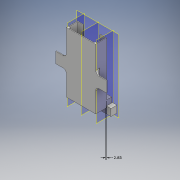
# Autodesk Inventor part: battery_case_1
Saved by Autodesk Inventor 2018 (Build 220112000, 112)
## iProperties
Created: 2019-07-20
Part Number: battery_case_1
Material: 一般
Document SubType Name: Modeling
Designer: guest1
Density: 1 g/cm^3
Appearance: 既定
Author: guest1
Autodesk Inventor part; units mm, degrees
ref_plane "YZ Plane" through (0, 0, 0) normal (1, 0, 0) x (0, 1, 0)
sketch "スケッチ1" plane through (0, 0, 0) normal (0, 0, 1) x (1, 0, 0)
  line L0 (-42.125, -17.075) -> (42.125, -17.075)
  line L1 (42.125, -17.075) -> (42.125, 15.125)
  line L2 (42.125, 15.125) -> (-42.125, 15.125)
  line L3 (-42.125, 15.125) -> (-42.125, -17.075)
  point P0 (0, 0)
  dimension "d0" = 84.25
  dimension "d1" = 32.2
  dimension "d140" = 15.125
  constraints: 8 end point, 2 parallel, 1 horizontal, 1 perpendicular
  measures "d0" distance of L1.end L2.end
  measures "d1" distance of L2.end L0.start
  measures "d140" distance from line of point (0, 0) L2
extrude "本体＿側" add sketch "スケッチ1" against normal blind 174
sketch "スケッチ3" plane through (0, 0, 0) normal (0, 0, 1) x (1, 0, 0)
  line L0 (-40.125, -12.075) -> (40.125, -12.075)
  line L1 (40.125, -12.075) -> (40.125, 13.125)
  line L2 (40.125, 13.125) -> (-40.125, 13.125)
  line L3 (-40.125, 13.125) -> (-40.125, -12.075)
  line L4 (42.125, 15.125) -> (-42.125, 15.125) projected
  line L5 (-42.125, -17.075) -> (42.125, -17.075) projected
  line L6 (-42.125, 15.125) -> (-42.125, -17.075) projected
  dimension "d4" = 80.25
  dimension "d125" = 2
  dimension "d138" = 2
  dimension "d139" = 25.2
  constraints: 8 end point, 2 parallel, 1 horizontal, 1 perpendicular
  measures "d4" distance of L1.end L2.end
  measures "d125" distance from line of L4 L2.end
  measures "d138" distance between parallel lines of L6 L3
  measures "d139" distance of L2.end L0.start
extrude "本体" cut sketch "スケッチ3" against normal blind 170
sketch "スケッチ6" plane through (0, 0, -174) normal (0, 0, -1) x (-1, 0, 0)
  line L0 (55, 48.1251) -> (-55, 48.1251)
  line L1 (-55, 48.1251) -> (-55, 14.1251)
  line L2 (-55, 14.1251) -> (55, 14.1251)
  line L3 (55, 14.1251) -> (55, 48.1251)
  line L4 (55, 48.1251) -> (-55, 14.1251) construction
  line L5 (-55, 48.1251) -> (55, 14.1251) construction
  line L6 (0, 0) -> (0, 97.4837)
  point P0 (0, 31.1251)
  point P1 (0, 31.1251)
  dimension "d8" = 110
  dimension "d9" = 34
  constraints: 14 end point, 3 midpoint, 3 parallel, 1 horizontal, 1 perpendicular, 1 point on line
  measures "d8" distance of L0.start L0.end
  measures "d9" distance of L0.end L1.end
extrude "カメラ" add sketch "スケッチ6" along normal blind 15.5 and the other way blind 4.5
sketch "スケッチ7" plane through (0, 0, -189.5) normal (0, 0, -1) x (-1, 0, 0)
  line L0 (-55, 48.1251) -> (-55, 14.1251) projected
  line L1 (-53, 16.1124) -> (53, 16.1124)
  line L2 (53, 16.1124) -> (53, 46.2624)
  line L3 (53, 46.2624) -> (-53, 46.2624)
  line L4 (-53, 46.2624) -> (-53, 16.1124)
  line L5 (-53, 16.1124) -> (53, 46.2624) construction
  line L6 (53, 16.1124) -> (-53, 46.2624) construction
  point P0 (0, 0)
  point P1 (-55, 31.1251)
  point P2 (-55, 31.1251)
  point P3 (0, 31.1874)
  point P4 (0, 31.1874)
  dimension "d14" = 30.15
  dimension "d15" = 106
  constraints: 12 end point, 4 midpoint, 2 parallel, 1 coincident, 1 horizontal, 1 perpendicular, 1 other
  measures "d14" distance of L1.end L2.end
  measures "d15" distance of L2.end L3.end
extrude "カメラ＿本体" cut sketch "スケッチ7" against normal blind 18
ref_plane "作業平面1" through (-55, 31.1251, -189.5) normal (0, 1, 0) x (1, 0, 0)
ref_plane "作業平面2" through (0, 14.1251, -189.5) normal (-1, 0, 0) x (0, 0, 1)
sketch "スケッチ10" plane through (-53, 16.1124, -189.5) normal (0, 1, 0) x (1, 0, 0)
  line L0 (59.8, -12.45) -> (46.2, -12.45)
  line L1 (46.2, -12.45) -> (46.2, 0)
  line L2 (46.2, 0) -> (59.8, 0)
  line L3 (59.8, 0) -> (59.8, -12.45)
  line L4 (59.8, -12.45) -> (46.2, 0) construction
  line L5 (46.2, -12.45) -> (59.8, 0) construction
  line L6 (108, -20) -> (-2, -20)
  line L7 (53, -20) -> (53, -4.9349)
  line L8 (53, -227.4) -> (53, 37.9)
  line L9 (0, 0) -> (106, 0)
  line L10 (0, 0) -> (106, 0)
  line L11 (0, 0) -> (0, -18)
  line L12 (0, -18) -> (106, -18)
  line L13 (106, 0) -> (106, -18)
  point P0 (53, -189.5)
  point P1 (53, -6.225)
  point P2 (53, 0)
  dimension "d22" = 12.45
  dimension "d23" = 13.6
  constraints: 28 end point, 4 midpoint, 1 point on line
  measures "d22" distance of L0.end L1.end
  measures "d23" distance of L0.start L0.end
sketch "スケッチ11" plane through (0, 0, -169.5) normal (0, 0, 1) x (1, 0, 0)
  line L0 (-15, 22.8501) -> (15, 22.8501)
  line L1 (15, 22.8501) -> (15, 39.4001)
  line L2 (15, 39.4001) -> (-15, 39.4001)
  line L3 (-15, 39.4001) -> (-15, 22.8501)
  line L4 (-53, 31.1251) -> (53, 31.1251)
  line L5 (-15, 22.8501) -> (15, 39.4001) construction
  line L6 (15, 22.8501) -> (-15, 39.4001) construction
  line L7 (0, -24.4525) -> (0, 47.8399)
  point P0 (0, 0)
  point P1 (0, 31.1251)
  point P2 (0, 31.1251)
  dimension "d26" = 30
  dimension "d27" = 16.55
  constraints: 16 end point, 4 midpoint, 1 point on line
  measures "d26" distance of L1.end L2.end
  measures "d27" distance of L2.end L0.start
extrude "突起" cut sketch "スケッチ10" against normal blind 2 contours L0 L7 L8 L2 L3 | L0 L1 L2 L8 L7
extrude "コード" cut sketch "スケッチ11" against normal blind 2
ref_plane "作業平面6" through (53, 16.1124, -189.5) normal (0, 0, 1) x (1, 0, 0)
sketch "スケッチ18" plane through (53, 16.1124, -189.5) normal (0, 0, 1) x (1, 0, 0)
  line L0 (0, 0) -> (0, 30.15) projected
  ellipse E0 centre (0, 15.0748) end of major axis (0, 0) minor radius 3.8117 (0, 30.1495) -> (0, 0) ccw
  line L1 (0, 30.15) -> (-106, 30.15) projected
  line L2 (-106, 0) -> (0, 0) projected
  line L3 (0, 30.15) -> (0, 0)
  point P0 (-53, -16.1124)
  constraints: 3 end point, 2 point on line, 2 vertical, 4 other
extrude "半円１" add sketch "スケッチ18" along normal blind 2
sketch "スケッチ19" plane through (53, 16.1124, -189.5) normal (0, 0, 1) x (1, 0, 0)
  line L0 (-106, 30.15) -> (-106, 0) projected
  ellipse E0 centre (-106.01, 15.0751) end of major axis (-106.0154, 30.1501) minor radius 3.8117 (-106.01, 0) -> (-106.01, 30.1501) ccw
  line L1 (-38, 6.7377) -> (-38, 23.2877) projected
  line L2 (-38, 23.2877) -> (-68, 23.2877) projected
  line L3 (-68, 23.2877) -> (-68, 6.7377) projected
  line L4 (-68, 6.7377) -> (-38, 6.7377) projected
  line L5 (-106, 0) -> (0, 0) projected
  line L6 (-106, 30.15) -> (-106, 0) projected
  line L7 (0, 30.15) -> (-106, 30.15) projected
  line L8 (0, 0) -> (0, 30.15) projected
  line L9 (-106, 0) -> (0, 0) projected
  line L10 (0, 30.15) -> (-106, 30.15) projected
  line L11 (-106, 0) -> (-106, 30.15)
  point P0 (-53, -16.1124)
  constraints: 2 end point, 1 perpendicular, 6 other
extrude "半円2" add sketch "スケッチ19" along normal blind 2 contours E0 L0
sketch "スケッチ16" plane through (-55, 31.1251, -189.5) normal (0, 1, 0) x (1, 0, 0)
  line L0 (110, -20) -> (110, 0) projected
  line L1 (0, -20) -> (0, 0) projected
  line L2 (110, 0) -> (0, 0)
  line L3 (0, 0) -> (0, -20)
  line L4 (0, -20) -> (110, -20)
  line L5 (110, -20) -> (110, 0)
  point P0 (55, -189.5)
  constraints: 8 end point, 2 parallel, 1 horizontal, 1 perpendicular
extrude "上半分消去" cut sketch "スケッチ16" along normal blind 17
sketch "スケッチ20" plane through (-42.125, 15.125, 0) normal (0, 1, 0) x (1, 0, 0)
  line L0 (18, 0) -> (66.25, 0)
  line L1 (66.25, 0) -> (66.25, 170)
  line L2 (66.25, 170) -> (18, 170)
  line L3 (18, 170) -> (18, 0)
  line L4 (18, 0) -> (66.25, 170) construction
  line L5 (66.25, 0) -> (18, 170) construction
  line L6 (84.25, 0) -> (0, 0) projected
  line L7 (42.125, -37.9) -> (42.125, 227.4) projected
  point P0 (42.125, 85)
  point P1 (42.125, 0)
  point P2 (42.125, 85)
  dimension "d47" = 170
  dimension "d91" = 18
  constraints: 12 end point, 5 midpoint, 3 coincident, 2 parallel, 1 horizontal, 1 perpendicular, 1 point on line
  measures "d47" distance of L2.end L0.start
  measures "d91" distance of L6.start L0.end
extrude "ボタン部" cut sketch "スケッチ20" against normal blind 2
ref_plane "作業平面7" through (-42.125, 15.125, 0) normal (-1, 0, 0) x (0, 0, -1)
sketch "スケッチ22" plane through (-42.125, 15.125, 0) normal (-1, 0, 0) x (0, 0, -1)
  line L0 (0, 0) -> (174, 0) projected
  line L1 (169.5, 0) -> (154.5, 0)
  line L2 (154.5, 0) -> (154.5, -14)
  line L3 (154.5, -14) -> (169.5, -14)
  line L4 (169.5, -14) -> (169.5, 0)
  point P0 (0, 15.125)
  point P1 (169.5, 0.9999)
  dimension "d51" = 15
  dimension "d52" = 14
  constraints: 8 end point, 2 parallel, 2 point on line, 1 horizontal, 1 perpendicular
  measures "d51" distance of L2.end L3.end
  measures "d52" distance of L1.end L2.end
extrude "支え１" add sketch "スケッチ22" against normal blind 15
ref_plane "作業平面8" through (42.125, 15.125, 0) normal (-1, 0, 0) x (0, 0, -1)
sketch "スケッチ23" plane through (42.125, 15.125, 0) normal (-1, 0, 0) x (0, 0, -1)
  line L0 (0, 0) -> (174, 0) projected
  line L1 (154.5, -14) -> (154.5, 0) projected
  line L2 (169.5, 0) -> (154.5, 0)
  line L3 (154.5, 0) -> (154.5, -14)
  line L4 (154.5, -14) -> (169.5, -14)
  line L5 (169.5, -14) -> (169.5, 0)
  point P0 (0, 15.125)
  dimension "d55" = 15
  dimension "d56" = 14
  constraints: 8 end point, 2 parallel, 1 horizontal, 1 perpendicular, 1 point on line
  measures "d55" distance of L1.start L4.end
  measures "d56" distance of L1.start L1.end
extrude "支え２" add sketch "スケッチ23" along normal blind 15
ref_plane "作業平面9" through (42.125, -17.075, 0) normal (0, 0, 1) x (0, 1, 0)
sketch "スケッチ24" plane through (42.125, -17.075, 0) normal (0, 0, 1) x (0, 1, 0)
  line L0 (0, 84.25) -> (31.2001, 84.25) projected
  line L1 (0, 0) -> (0, 84.25) projected
  line L2 (28.25, 84.25) -> (0, 84.25)
  line L3 (0, 84.25) -> (0, 0)
  line L4 (0, 0) -> (28.25, 0)
  line L5 (28.25, 0) -> (28.25, 84.25)
  point P0 (17.075, 42.125)
  constraints: 8 end point, 2 parallel, 1 horizontal, 1 perpendicular
extrude "削除予定" [suppressed]
sketch "スケッチ43" plane through (0, 0, 0) normal (0, 0, 1) x (1, 0, 0)
  line L0 (40.125, -12.075) -> (-40.125, -12.075) projected
  line L1 (0, -12.075) -> (31, -12.075)
  line L2 (26.4993, -15.075) -> (26.4993, -12.075)
  line L3 (26.4993, -12.075) -> (35.4993, -12.075)
  line L4 (35.4993, -12.075) -> (35.4993, -15.075)
  line L5 (35.4993, -15.075) -> (26.4993, -15.075)
  line L6 (26.4993, -15.075) -> (35.4993, -12.075) construction
  line L7 (26.4993, -12.075) -> (35.4993, -15.075) construction
  line L8 (30.9993, -12.075) -> (30.9993, -17.075)
  line L9 (-42.125, -17.075) -> (42.125, -17.075) projected
  point P0 (0, 0)
  point P1 (31, -12.125)
  dimension "d127" = 31
  dimension "d128" = 3
  dimension "d130" = 9
  constraints: 16 end point, 3 point on line, 2 midpoint, 2 parallel, 2 vertical, 1 perpendicular
  measures "d127" distance of L1.start L1.end
  measures "d128" distance of L2.start L2.end
  measures "d130" distance of L4.end L2.start
extrude "ネジ山溝１" cut sketch "スケッチ43" against normal blind 170
sketch "スケッチ44" plane through (0, 0, 0) normal (0, 0, 1) x (1, 0, 0)
  line L0 (26.4993, -12.075) -> (-40.125, -12.075) projected
  line L1 (0, -12.075) -> (-31, -12.075)
  line L2 (0, -30.115) -> (0, 61.1651) projected
  line L3 (-26.5, -15.075) -> (-26.5, -12.075)
  line L4 (-26.5, -12.075) -> (-35.5, -12.075)
  line L5 (-35.5, -12.075) -> (-35.5, -15.075)
  line L6 (-35.5, -15.075) -> (-26.5, -15.075)
  line L7 (-26.5, -15.075) -> (-35.5, -12.075) construction
  line L8 (-26.5, -12.075) -> (-35.5, -15.075) construction
  line L9 (-42.125, -17.075) -> (42.125, -17.075) projected
  line L10 (-31, -17.075) -> (-31, -12.075)
  point P0 (0, 0)
  point P1 (-31, -13.575)
  point P2 (-31, -13.575)
  dimension "d133" = 31
  dimension "d134" = 9
  dimension "d135" = 3
  constraints: 16 end point, 6 point on line, 3 midpoint, 2 parallel, 2 perpendicular, 1 vertical
  measures "d133" distance of L1.start L1.end
  measures "d134" distance of L5.end L3.start
  measures "d135" distance of L4.end L5.end
extrude "ネジ山溝２" cut sketch "スケッチ44" against normal blind 170 contours L3 L6 L10 L0 | L10 L6 L5 L0
sketch "スケッチ47" plane through (42.125, -17.075, 0) normal (1, 0, 0) x (0, 0, -1)
  line L0 (0, 0) -> (174, 0) projected
  line L1 (75, 2) -> (106, 2)
  line L2 (106, 2) -> (106, 0)
  line L3 (106, 0) -> (75, 0)
  line L4 (75, 0) -> (75, 2)
  line L5 (174, 31.2001) -> (174, 0) projected
  point P0 (0, 17.075)
  dimension "d141" = 68
  dimension "d142" = 31
  dimension "d145" = 2
  constraints: 8 end point, 2 parallel, 1 horizontal, 1 perpendicular, 1 point on line
  measures "d141" distance between parallel lines of L2 L5
  measures "d142" distance of L1.start L1.end
  measures "d145" distance of L3.end L1.start
extrude "押し出し28" add sketch "スケッチ47" along normal blind 31
sketch "スケッチ48" plane through (42.125, -15.075, -75) normal (0, 1, 0) x (1, 0, 0)
  point P0 (-42.125, -75)
fillet "フィレット1" radius 10 1 edges at (42.125, -15.075, -90.5)
fillet "フィレット2" radius 10 1 edges at (42.125, -16.075, -106)
fillet "フィレット3" radius 10 1 edges at (42.125, -16.075, -75)
sketch "スケッチ49" plane through (-42.125, -17.075, 0) normal (-1, 0, 0) x (0, 0, 1)
  line L0 (0, 0) -> (-174, 0) projected
  line L1 (-106, 0) -> (-75, 0)
  line L2 (-75, 0) -> (-75, 2)
  line L3 (-75, 2) -> (-106, 2)
  line L4 (-106, 2) -> (-106, 0)
  line L5 (-174, 0) -> (-174, 31.2001) projected
  point P0 (0, 17.075)
  dimension "d149" = 68
  dimension "d150" = 31
  dimension "d151" = 2
  constraints: 8 end point, 2 parallel, 1 horizontal, 1 perpendicular, 1 point on line
  measures "d149" distance between parallel lines of L4 L5
  measures "d150" distance of L2.end L3.end
  measures "d151" distance of L1.end L2.end
extrude "押し出し29" add sketch "スケッチ49" along normal blind 31
fillet "フィレット4" radius 10 1 edges at (-42.125, -15.075, -90.5)
fillet "フィレット5" radius 10 1 edges at (-42.125, -16.075, -75)
fillet "フィレット6" radius 10 1 edges at (-42.125, -16.075, -106)
sketch "スケッチ56" plane through (0, 0, 0) normal (0, 0, 1) x (1, 0, 0)
  line L0 (26.4993, -12.075) -> (-26.5, -12.075) projected
  line L1 (35.4993, -15.075) -> (26.4993, -15.075) projected
  line L2 (-26.5, -12.075) -> (26.4993, -12.075)
  line L3 (26.4993, -12.075) -> (26.4993, -15.075)
  line L4 (26.4993, -15.075) -> (-26.5, -15.075)
  line L5 (-26.5, -15.075) -> (-26.5, -12.075)
  point P0 (0, 0)
  constraints: 8 end point, 2 parallel, 1 horizontal, 1 perpendicular
extrude "キャスターネジ溝" cut sketch "スケッチ56" against normal blind 35
